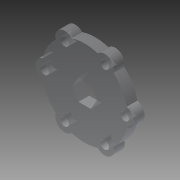
# Autodesk Inventor part: Custom Belt Pulley Hex Hub (polycarbonate)
Saved by Autodesk Inventor 2013 (Build 170138000, 138)
## iProperties
Created: 2013-01-17
Part Number: Custom Belt Pulley Hex Hub (polycarbonate)
Material: Polycarbonate, Clear
Document SubType Name: Modeling
Designer: Moses
Density: 0.894 g/cm^3
Mass: 8.44161 g
Surface Area: 55.1406 cm^2
Volume: 9.44251 cm^3
Author: Moses
Autodesk Inventor part; units mm, degrees
ref_plane "YZ Plane" through (0, 0, 0) normal (1, 0, 0) x (0, 1, 0)
ref_plane "XZ Plane" through (0, 0, 0) normal (0, 1, 0) x (-1, 0, 0)
ref_plane "XY Plane" through (0, 0, 0) normal (0, 0, 1) x (1, 0, 0)
sketch "Sketch1" plane through (0, 0, 0) normal (0, 0, 1) x (1, 0, 0)
  arc A0 (-7.8064, 24.3719) -> (-17.2043, 18.9457) centre (-11.9071, 20.6227) ccw projected
  arc A1 (-17.2043, 18.9457) -> (-20.4582, 15.375) centre (0, 0) ccw projected
  arc A2 (-17.7043, 15.4859) -> (-20.4582, 15.375) centre (-19.036, 14.3062) ccw construction
  arc A3 (-17.7043, 15.4859) -> (-14.4866, 13.3187) centre (-11.9063, 20.6222) ccw construction
  arc A4 (-13.671, 10.5541) -> (-14.4866, 13.3187) centre (-15.0792, 11.6413) ccw construction
  arc A5 (-13.671, 10.5541) -> (-15.9756, 6.5626) centre (0, 0) ccw construction
  arc A6 (-18.7774, 5.8865) -> (-15.9756, 6.5626) centre (-17.6212, 7.2386) ccw construction
  arc A7 (-18.7774, 5.8865) -> (-22.2633, 7.5891) centre (-23.8116, -0.0005) ccw construction
  arc A8 (-23.5444, 10.0295) -> (-22.2633, 7.5891) centre (-21.9076, 9.3323) ccw construction
  arc A9 (-23.5444, 10.0295) -> (-25.0098, 5.4257) centre (0, 0) ccw projected
  arc A10 (-25.0098, 5.4257) -> (-25.0098, -5.4257) centre (-23.8125, 0) ccw projected
  arc A11 (-25.0098, -5.4257) -> (-23.5442, -10.0298) centre (0, 0) ccw projected
  arc A12 (-22.2633, -7.5894) -> (-23.5442, -10.0298) centre (-21.9075, -9.3326) ccw construction
  arc A13 (-22.2633, -7.5894) -> (-18.7776, -5.8864) centre (-23.8125, 0) ccw construction
  arc A14 (-15.9756, -6.5624) -> (-18.7776, -5.8864) centre (-17.6212, -7.2384) ccw construction
  arc A15 (-15.9756, -6.5624) -> (-13.6711, -10.554) centre (0, 0) ccw construction
  arc A16 (-14.4865, -13.3185) -> (-13.6711, -10.554) centre (-15.0794, -11.6411) ccw construction
  arc A17 (-14.4865, -13.3185) -> (-17.704, -15.486) centre (-11.9054, -20.6217) ccw construction
  arc A18 (-20.458, -15.3753) -> (-17.704, -15.486) centre (-19.0358, -14.3064) ccw construction
  arc A19 (-20.458, -15.3753) -> (-17.2032, -18.9467) centre (0, 0) ccw projected
  arc A20 (-17.2032, -18.9467) -> (-7.8058, -24.3721) centre (-11.9054, -20.6217) ccw projected
  arc A21 (-7.8058, -24.3721) -> (-3.0861, -25.4048) centre (0, 0) ccw projected
  arc A22 (-4.559, -23.0753) -> (-3.0861, -25.4048) centre (-2.8715, -23.6387) ccw construction
  arc A23 (-4.559, -23.0753) -> (-4.291, -19.2051) centre (-11.9062, -20.6222) ccw construction
  arc A24 (-2.3046, -17.1165) -> (-4.291, -19.2051) centre (-2.542, -18.8796) ccw construction
  arc A25 (-2.3046, -17.1165) -> (2.3044, -17.1165) centre (0, 0) ccw construction
  arc A26 (4.2909, -19.2049) -> (2.3044, -17.1165) centre (2.5418, -18.8797) ccw construction
  arc A27 (4.2909, -19.2049) -> (4.5593, -23.0751) centre (11.9062, -20.6212) ccw construction
  arc A28 (3.0864, -25.4048) -> (4.5593, -23.0751) centre (2.8718, -23.6387) ccw construction
  arc A29 (3.0864, -25.4048) -> (7.8078, -24.3714) centre (0, 0) ccw projected
  arc A30 (7.8078, -24.3714) -> (17.2047, -18.9453) centre (11.9071, -20.6207) ccw projected
  arc A31 (17.2047, -18.9453) -> (20.4582, -15.375) centre (0, 0) ccw projected
  arc A32 (17.7043, -15.4859) -> (20.4582, -15.375) centre (19.036, -14.3062) ccw construction
  arc A33 (17.7043, -15.4859) -> (14.4866, -13.3187) centre (11.9063, -20.6222) ccw construction
  arc A34 (13.671, -10.5541) -> (14.4866, -13.3187) centre (15.0792, -11.6413) ccw construction
  arc A35 (13.671, -10.5541) -> (15.9756, -6.5626) centre (0, 0) ccw construction
  arc A36 (18.7774, -5.8865) -> (15.9756, -6.5626) centre (17.6212, -7.2386) ccw construction
  arc A37 (18.7774, -5.8865) -> (22.2633, -7.5891) centre (23.8116, 0.0005) ccw construction
  arc A38 (23.5444, -10.0295) -> (22.2633, -7.5891) centre (21.9076, -9.3323) ccw construction
  arc A39 (23.5444, -10.0295) -> (25.0102, -5.4236) centre (0, 0) ccw projected
  arc A40 (25.0102, -5.4236) -> (25.0093, 5.4278) centre (23.8125, 0.002) ccw projected
  arc A41 (25.0093, 5.4278) -> (23.5442, 10.0298) centre (0, 0) ccw projected
  arc A42 (22.2633, 7.5894) -> (23.5442, 10.0298) centre (21.9075, 9.3326) ccw construction
  arc A43 (22.2633, 7.5894) -> (18.7776, 5.8864) centre (23.8125, 0) ccw construction
  arc A44 (15.9756, 6.5624) -> (18.7776, 5.8864) centre (17.6212, 7.2384) ccw construction
  arc A45 (15.9756, 6.5624) -> (13.6711, 10.554) centre (0, 0) ccw construction
  arc A46 (14.4865, 13.3185) -> (13.6711, 10.554) centre (15.0794, 11.6411) ccw construction
  arc A47 (14.4865, 13.3185) -> (17.704, 15.486) centre (11.9054, 20.6217) ccw construction
  arc A48 (20.458, 15.3753) -> (17.704, 15.486) centre (19.0358, 14.3064) ccw construction
  arc A49 (20.458, 15.3753) -> (17.2027, 18.9472) centre (0, 0) ccw projected
  arc A50 (17.2027, 18.9472) -> (7.8044, 24.3725) centre (11.9054, 20.6237) ccw projected
  arc A51 (7.8044, 24.3725) -> (3.0861, 25.4048) centre (0, 0) ccw projected
  arc A52 (4.559, 23.0753) -> (3.0861, 25.4048) centre (2.8715, 23.6387) ccw construction
  arc A53 (4.559, 23.0753) -> (4.291, 19.2051) centre (11.9062, 20.6222) ccw construction
  arc A54 (2.3046, 17.1165) -> (4.291, 19.2051) centre (2.542, 18.8796) ccw construction
  arc A55 (2.3046, 17.1165) -> (-2.3044, 17.1165) centre (0, 0) ccw construction
  arc A56 (-4.2909, 19.2049) -> (-2.3044, 17.1165) centre (-2.5418, 18.8797) ccw construction
  arc A57 (-4.2909, 19.2049) -> (-4.5593, 23.0751) centre (-11.9062, 20.6212) ccw construction
  arc A58 (-3.0864, 25.4048) -> (-4.5593, 23.0751) centre (-2.8718, 23.6387) ccw construction
  arc A59 (-3.0864, 25.4048) -> (-7.8064, 24.3719) centre (0, 0) ccw projected
  circle A60 centre (-11.9071, 20.6227) radius 2.54 projected
  circle A61 centre (11.9054, 20.6237) radius 2.54 projected
  circle A62 centre (23.8125, 0.002) radius 2.54 projected
  circle A63 centre (11.9071, -20.6207) radius 2.54 projected
  circle A64 centre (-11.9054, -20.6217) radius 2.54 projected
  circle A65 centre (-23.8125, 0) radius 2.54 projected
  circle A66 centre (0, 0) radius 14.2875 construction
  arc A67 (-20.4582, 15.375) -> (-23.5444, 10.0295) centre (0, 0) ccw
  line L0 (7.3323, 0) -> (3.6662, -6.35)
  line L1 (3.6662, -6.35) -> (-3.6662, -6.35)
  line L2 (-3.6662, -6.35) -> (-7.3323, 0)
  line L3 (-7.3323, 0) -> (-3.6662, 6.35)
  line L4 (-3.6662, 6.35) -> (3.6662, 6.35)
  line L5 (3.6662, 6.35) -> (7.3323, 0)
  line L6 (0, 0) -> (7.3323, 0) construction
  arc A68 (3.0861, 25.4048) -> (-3.0864, 25.4048) centre (0, 0) ccw
  arc A69 (23.5442, 10.0298) -> (20.458, 15.3753) centre (0, 0) ccw
  arc A70 (20.4582, -15.375) -> (23.5444, -10.0295) centre (0, 0) ccw
  arc A71 (-3.0861, -25.4048) -> (3.0864, -25.4048) centre (0, 0) ccw
  arc A72 (-23.5442, -10.0298) -> (-20.458, -15.3753) centre (0, 0) ccw
  point P0 (0, 0)
  dimension "d0" = 12.7
  constraints: 14 end point, 12 point on circle, 6 centre point, 6 concentric, 2 coincident, 1 horizontal, 1 parallel, 13 other
  measures "d0" distance between parallel lines of L1 L4
extrude "Extrusion1" add sketch "Sketch1" along normal blind 6.35
body "Solid1"
